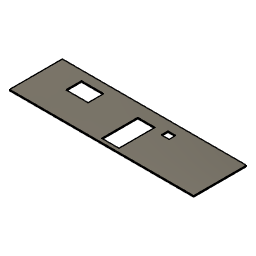
Bauwagen Seite lang Deichsel rechts v2 (Autodesk Fusion 360 design; units mm, degrees)
Autodesk Fusion 360 part; units mm, degrees
note: some values were not read from the file. Set by a fixed rule: which sketch regions a step uses.
sketch "Skizze1" plane through (0, 0, 0) normal (0, 1, 0) x (1, 0, 0)
  line L0 (0, 0) -> (827, 0)
  line L1 (827, 0) -> (827, -195)
  line L2 (827, -195) -> (0, -195)
  line L3 (0, -195) -> (0, 0)
  line L4 (0, -195) -> (128, -195)
  line L5 (128, -195) -> (128, -70)
  line L6 (128, -70) -> (228, -70)
  line L7 (228, -70) -> (228, 0)
  line L8 (228, 0) -> (128, 0)
  line L9 (128, 0) -> (128, -70)
  dimension "d1" = 827
  dimension "d2" = 195
  dimension "d3" = 128
  dimension "d4" = 125
  dimension "d5" = 100
  dimension "d6" = 70
  constraint horizontal L0
  constraint vertical L1
  constraint horizontal L2
  constraint vertical L3
  constraint coincident L0.start L3.end
  constraint perpendicular L3 L4
  constraint perpendicular L2 L5
  constraint horizontal L6
  constraint vertical L7
  constraint horizontal L8
  constraint vertical L9
  measures "d1" distance of L0.start L0.end
  measures "d2" distance of L0.start L2.end
  measures "d3" distance of L2.end L4.end
  measures "d4" distance of L4.end L5.end
  measures "d5" distance of L5.end L6.end
  measures "d6" distance of L5.end L8.end
extrude "Extrusion1" add sketch "Skizze1" along normal blind 5 contours L0 L2 L3 L4 L5 L9 | L0 L1 L2 L5 L6 L7
extrude "Extrusion2" add 2 faces at (427.6667, 1.6667, 0) (42.6667, 3.3333, 0) along direction (0, 0, -1) blind 1
sketch "Skizze2" plane through (0, 5, 0) normal (0, 1, 0) x (-1, 0, 0)
  line L0 (0, 195) -> (-827, 195)
  line L1 (-827, 195) -> (-827, -1)
  line L2 (-827, -1) -> (-228, -1)
  line L3 (-228, -1) -> (-228, 70)
  line L4 (-228, 70) -> (-128, 70)
  line L5 (-128, 70) -> (-128, -1)
  line L6 (-128, -1) -> (0, -1)
  line L7 (0, -1) -> (0, 195)
  line L8 (-128, -1) -> (-228, -1)
  line L9 (-128, -1) -> (-128, 0)
  line L10 (-128, 0) -> (-228, 0)
  line L11 (-228, -1) -> (-228, 0)
  constraint coincident L5.end L6.start
  constraint coincident L2.end L3.start
  constraint coincident L5 L9.end
  constraint coincident L3 L10.end
  constraint perpendicular L3 L10
extrude "Extrusion3" add sketch "Skizze2" against normal blind 5 contours L3 L5 L8 L9 L10 L11
sketch "Skizze3" plane through (0, 5, 0) normal (0, 1, 0) x (-1, 0, 0)
  line L0 (-228, 0) -> (-228, 70)
  line L1 (-228, 70) -> (-128, 70)
  line L2 (-128, 70) -> (-128, 0)
  line L3 (-128, 0) -> (-228, 0)
  line L4 (-827, -1) -> (0, -1)
  line L5 (0, -1) -> (0, 195)
  line L6 (0, 195) -> (-827, 195)
  line L7 (-827, 195) -> (-827, -1)
  line L8 (0, 195) -> (-354, 195)
  line L9 (-354, 195) -> (-354, 178)
  line L10 (-354, 178) -> (-431.5, 178)
  line L11 (-431.5, 178) -> (-431.5, 16)
  line L12 (-431.5, 16) -> (-354, 16)
  line L13 (-354, 16) -> (-354, 178)
  dimension "d13" = 354
  dimension "d14" = 17
  dimension "d15" = 77.5
  dimension "d16" = 162
  constraint coincident L5.end L6.start
  constraint perpendicular L5 L8
  constraint perpendicular L6 L9
  constraint horizontal L10
  constraint vertical L11
  constraint horizontal L12
  constraint vertical L13
  measures "d13" distance of L5.end L8.end
  measures "d14" distance of L8.end L9.end
  measures "d15" distance of L9.end L10.end
  measures "d16" distance of L9.end L12.end
extrude "Extrusion4" cut sketch "Skizze3" against normal blind 5 contours L10 L11 L12 L13
sketch "Skizze4" plane through (0, 5, 0) normal (0, 1, 0) x (-1, 0, 0)
  line L0 (-431.5, 178) -> (-354, 178)
  line L1 (-354, 178) -> (-354, 16)
  line L2 (-354, 16) -> (-431.5, 16)
  line L3 (-228, 0) -> (-228, 70)
  line L4 (-228, 70) -> (-128, 70)
  line L5 (-128, 70) -> (-128, 0)
  line L6 (-128, 0) -> (-228, 0)
  line L7 (-827, -1) -> (0, -1)
  line L8 (0, -1) -> (0, 195)
  line L9 (0, 195) -> (-827, 195)
  line L10 (-827, 195) -> (-827, -1)
  line L11 (-827, -1) -> (-531, -1)
  line L12 (-531, -1) -> (-531, 195)
  line L13 (-531, 195) -> (-531, 33)
  line L14 (-531, 33) -> (-496, 33)
  line L15 (-496, 33) -> (-496, 3)
  line L16 (-496, 3) -> (-531, 3)
  line L17 (-531, 3) -> (-531, 33)
  line L18 (-431.5, 16) -> (-474.5, 16)
  line L19 (-474.5, 16) -> (-397, 16)
  line L20 (-397, 16) -> (-397, 178)
  line L21 (-397, 178) -> (-474.5, 178)
  line L22 (-474.5, 178) -> (-474.5, 16)
  dimension "d19" = 296
  dimension "d20" = 162
  dimension "d21" = 35
  dimension "d22" = 30
  dimension "d23" = 43
  dimension "d24" = 162
  dimension "d25" = 77.5
  constraint coincident L7.start L10.end
  constraint perpendicular L10 L11
  constraint coincident L9 L12.end
  constraint perpendicular L9 L12
  constraint perpendicular L9 L13
  constraint horizontal L14
  constraint vertical L15
  constraint horizontal L16
  constraint vertical L17
  constraint coincident L2.end L18.start
  constraint horizontal L19
  constraint vertical L20
  constraint horizontal L21
  constraint vertical L22
  measures "d19" distance of L7.start L11.end
  measures "d20" distance of L12.end L13.end
  measures "d21" distance of L13.end L14.end
  measures "d22" distance of L13.end L16.end
  measures "d23" distance of L2.end L18.end
  measures "d24" distance of L18.end L21.end
  measures "d25" distance of L18.end L19.end
extrude "Extrusion5" add sketch "Skizze4" against normal blind 5 contours L0 L1 L2 L20
sketch "Skizze5" plane through (0, 5, 0) normal (0, 1, 0) x (-1, 0, 0)
extrude "Extrusion6" cut sketch "Skizze4" against normal blind 40 contours L0 L2 L18 L19 L20 L21 L22
sketch "Skizze6" plane through (0, 5, 0) normal (0, 1, 0) x (-1, 0, 0)
  line L0 (-827, -1) -> (0, -1)
  line L1 (0, -1) -> (0, 195)
  line L2 (0, 195) -> (-827, 195)
  line L3 (-827, 195) -> (-827, -1)
  line L4 (-228, 0) -> (-228, 70)
  line L5 (-228, 70) -> (-128, 70)
  line L6 (-128, 70) -> (-128, 0)
  line L7 (-128, 0) -> (-228, 0)
  line L8 (-397, 16) -> (-474.5, 16)
  line L9 (-474.5, 16) -> (-474.5, 178)
  line L10 (-474.5, 178) -> (-397, 178)
  line L11 (-397, 178) -> (-397, 16)
  line L12 (-474.5, 16) -> (-517.5, 16)
  line L13 (-827, 195) -> (-827, 31)
  line L14 (-827, 31) -> (-474.5, 31)
  line L15 (-517.5, 16) -> (-517.5, 31)
  line L16 (-517.5, 31) -> (-552.5, 31)
  line L17 (-552.5, 31) -> (-552.5, 1)
  line L18 (-552.5, 1) -> (-517.5, 1)
  line L19 (-517.5, 1) -> (-517.5, 31)
  dimension "d30" = 43
  dimension "d31" = 164
  dimension "d32" = 35
  dimension "d33" = 30
  constraint horizontal L12
  constraint coincident L2.end L3.start
  constraint perpendicular L2 L13
  constraint coincident L9 L14.end
  constraint perpendicular L9 L14
  constraint coincident L14 L15.end
  constraint perpendicular L14 L15
  constraint horizontal L16
  constraint vertical L17
  constraint horizontal L18
  constraint vertical L19
  measures "d30" distance of L8.end L12.end
  measures "d31" distance of L2.end L13.end
  measures "d32" distance of L15.end L16.end
  measures "d33" distance of L15.end L18.end
extrude "Extrusion7" cut sketch "Skizze6" against normal blind 50 contours L14 L15 L16 L17 L18 L19
extrude "Extrusion8" add 1 faces at (275.6667, 3.3333, -1) along direction (0, 0, -1) blind 41
